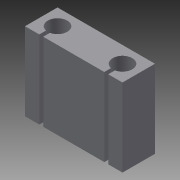
# Autodesk Inventor part: ChimeraXCarriage
Saved by Autodesk Inventor 2015 (Build 190159000, 159)
## iProperties
Created: 2014-11-29
Part Number: ChimeraXCarriage
Material: Generic
Document SubType Name: Modeling
Designer: Jack
Density: 1 g/cm^3
Appearance: Default
Author: Jack
Autodesk Inventor part; units mm, degrees
ref_plane "YZ Plane" through (0, 0, 0) normal (1, 0, 0) x (0, 1, 0)
ref_plane "XZ Plane" through (0, 0, 0) normal (0, 1, 0) x (-1, 0, 0)
ref_plane "XY Plane" through (0, 0, 0) normal (0, 0, 1) x (1, 0, 0)
sketch "Sketch1" plane through (0, 0, 0) normal (0, 0, 1) x (1, 0, 0)
  arc A0 (1.5, -7.3485) -> (-1.5, -7.3485) centre (0, 0) ccw
  arc A1 (51.5, -7.3485) -> (48.5, -7.3485) centre (50, 0) ccw
  line L0 (-1.5, -12.5) -> (-12.5, -12.5)
  line L1 (-12.5, -12.5) -> (-12.5, 12.5)
  line L2 (-12.5, 12.5) -> (62.5, 12.5)
  line L3 (62.5, 12.5) -> (62.5, -12.5)
  line L4 (62.5, -12.5) -> (51.5, -12.5)
  line L5 (51.5, -12.5) -> (51.5, -7.3485)
  line L6 (48.5, -7.3485) -> (48.5, -12.5)
  line L7 (1.5, -12.5) -> (1.5, -7.3485)
  line L8 (-1.5, -12.5) -> (-1.5, -7.3485)
  line L9 (1.5, -12.5) -> (48.5, -12.5)
  dimension "d0" = 15
  dimension "d2" = 12.5
  dimension "d3" = 12.5
  dimension "d4" = 12.5
  dimension "d8" = 12.5
  dimension "d9" = 3
  dimension "d10" = 1.5
  dimension "d11" = 3
  dimension "d12" = 1.5
  dimension "d13" = 50
  constraints: 20 end point, 5 perpendicular, 4 point on circle, 3 horizontal, 2 centre point, 2 parallel, 2 point on line, 1 coincident, 1 equal radius, 1 horizontal alignment
  measures "d0" diameter of A0
  measures "d2" distance from line of L0 point (0, 0)
  measures "d3" distance from line of point (0, 0) L1
  measures "d4" distance from line of A1.centre L3
  measures "d8" distance from line of point (0, 0) L2
  measures "d9" distance between parallel lines of L7 L8
  measures "d10" distance from line of point (0, 0) L8
  measures "d11" distance between parallel lines of L5 L6
  measures "d12" distance from line of A1.centre L5
  measures "d13" distance of A0.centre A1.centre
extrude "Extrusion1" add sketch "Sketch1" along normal blind 60
body "Solid1"
